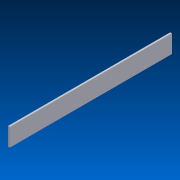
# Autodesk Inventor part: BOXC_F17P5
Saved by Autodesk Inventor 2012 (Build 160160000, 160)
## iProperties
Created: 2012-06-30
Part Number: BOXC_F17P5
Material: Default
Document SubType Name: Modeling
Designer: Hemant
Density: 1 g/cm^3
Author: Hemant
Autodesk Inventor part; units mm, degrees
ref_plane "YZ Plane" through (0, 0, 0) normal (1, 0, 0) x (0, 1, 0)
ref_plane "XZ Plane" through (0, 0, 0) normal (0, 1, 0) x (-1, 0, 0)
ref_plane "XY Plane" through (0, 0, 0) normal (0, 0, 1) x (1, 0, 0)
sketch "Sketch1" plane through (0, 0, 0) normal (0, 0, 1) x (1, 0, 0)
  line L0 (0, 50.8) -> (4.7625, 50.8)
  line L1 (4.7625, 50.8) -> (4.7625, 0)
  line L2 (4.7625, 0) -> (0, 0)
  line L3 (0, 0) -> (0, 50.8)
  dimension "d0" = 4.7625
  dimension "d1" = 50.8
  constraints: 8 end point, 2 parallel, 1 horizontal, 1 perpendicular
  measures "d0" distance between parallel lines of L1 L3
  measures "d1" distance between parallel lines of L0 L2
extrude "Extrusion1" add sketch "Sketch1" along normal blind 457.2
body "Solid1"
